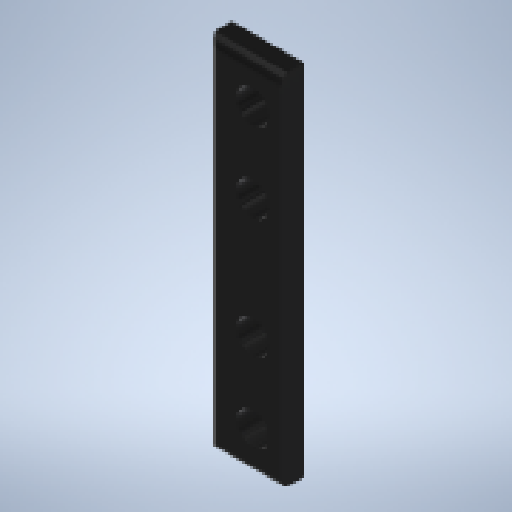
# Autodesk Inventor part: SMA_Spacer_AnalogConversion_v3
Saved by Autodesk Inventor 2023.1 (Build 271208000, 208)
## iProperties
Created: 2022-08-11
Part Number: SMA_Spacer_AnalogConversion_v3
Material: Generisch
Document SubType Name: Modeling
Designer: pd
Density: 1 g/cm^3
Appearance: Stahlblau - hell
Author: pd
Autodesk Inventor part; units mm, degrees
ref_plane "YZ Plane" through (0, 0, 0) normal (1, 0, 0) x (0, 1, 0)
ref_plane "XZ Plane" through (0, 0, 0) normal (0, 1, 0) x (-1, 0, 0)
sketch "Skizze1" plane through (0, 0, 0) normal (0, 0, 1) x (1, 0, 0)
  circle A0 centre (10.63, -52.2) radius 3.25 construction
  circle A1 centre (10.63, -76.2) radius 3.25 construction
  circle A2 centre (10.63, -36.2) radius 3.25 construction
  circle A3 centre (10.63, -92.2) radius 3.25 construction
  line L0 (19.98, -128.4) -> (0.8594, -128.4) construction
  line L1 (19.98, -128.4) -> (19.98, -114.2) construction
  line L2 (19.98, -114.2) -> (19.08, -114.2) construction
  line L3 (19.08, -114.2) -> (19.08, -14.2) construction
  line L4 (19.08, -14.2) -> (19.98, -14.2) construction
  line L5 (19.98, -14.2) -> (19.98, 0) construction
  line L6 (0.8594, 0) -> (19.98, 0) construction
  line L7 (0.8594, -14.2) -> (0.8594, 0) construction
  line L8 (0.8594, -14.2) -> (1.63, -14.2) construction
  line L9 (1.63, -114.2) -> (1.63, -14.2) construction
  line L10 (1.63, -114.2) -> (0.8594, -114.2) construction
  line L11 (0.8594, -128.4) -> (0.8594, -114.2) construction
  circle A4 centre (12.53, -14.7) radius 1.35 construction
  circle A5 centre (7.45, -113.7) radius 1.275 construction
  circle A6 centre (17.61, -113.7) radius 1.275 construction
  circle A7 centre (12.53, -113.7) radius 1.275 construction
  circle A8 centre (7.45, -3) radius 1.275 construction
  circle A9 centre (7.45, -125.4) radius 1.275 construction
  arc A10 (10.0846, -1.35) -> (10.0846, -4.65) centre (12.53, -3) ccw construction
  line L12 (14.9754, -1.35) -> (10.0846, -1.35) construction
  arc A11 (14.9754, -4.65) -> (14.9754, -1.35) centre (12.53, -3) ccw construction
  line L13 (10.0846, -4.65) -> (14.9754, -4.65) construction
  arc A12 (10.0846, -123.75) -> (10.0846, -127.05) centre (12.53, -125.4) ccw construction
  line L14 (14.9754, -123.75) -> (10.0846, -123.75) construction
  arc A13 (14.9754, -127.05) -> (14.9754, -123.75) centre (12.53, -125.4) ccw construction
  line L15 (10.0846, -127.05) -> (14.9754, -127.05) construction
  line L16 (16.13, -17.1308) -> (16.13, -111.2692) construction
  line L17 (1.63, -28.2) -> (16.13, -28.2)
  line L18 (16.13, -28.2) -> (16.13, -100.2)
  line L19 (16.13, -100.2) -> (1.63, -100.2)
  line L20 (1.63, -100.2) -> (1.63, -28.2)
  circle A14 centre (10.63, -36.2) radius 3.25
  circle A15 centre (10.63, -52.2) radius 3.25
  circle A16 centre (10.63, -76.2) radius 3.25
  circle A17 centre (10.63, -92.2) radius 3.25
  point P0 (0, 0)
  dimension "d0" = 0
  dimension "d1" = 0
  dimension "d2" = 8
  dimension "d3" = 8
  dimension "d4" = 6.5
  dimension "d5" = 6.5
  dimension "d6" = 6.5
  dimension "d7" = 6.5
  constraints: 8 end point, 4 centre point, 4 coincident, 2 parallel, 1 horizontal, 1 perpendicular
  measures "d0" distance between parallel lines of L9 L20
  measures "d1" distance between parallel lines of L16 L18
  measures "d2" distance from line of A2.centre L17
  measures "d3" distance from line of A3.centre L19
  measures "d4" diameter of A14
  measures "d5" diameter of A15
  measures "d6" diameter of A16
  measures "d7" diameter of A17
ref_plane "Arbeitsebene1" through (7.63, -39.2, 4.8) normal (0, 0, -1) x (0, 1, 0)
extrude "Extrusion1" add sketch "Skizze1" along normal up to surface (4.8 mm away)
fillet "Rundung1" radius 2 3 edges at (1.63, -64.2, 4.8) (8.88, -100.2, 4.8) (8.88, -28.2, 4.8)
